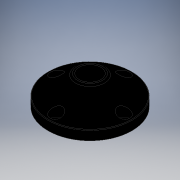
# Autodesk Inventor part: Base
Saved by Autodesk Inventor 2017 (Build 210142000, 142)
## iProperties
Created: 2020-05-28
Part Number: Base
Material: Generic
Document SubType Name: Modeling
Designer: Sid
Density: 1 g/cm^3
Appearance: Default
Author: Sid
Autodesk Inventor part; units mm, degrees
ref_plane "YZ Plane" through (0, 0, 0) normal (1, 0, 0) x (0, 1, 0)
ref_plane "XZ Plane" through (0, 0, 0) normal (0, 1, 0) x (-1, 0, 0)
ref_plane "XY Plane" through (0, 0, 0) normal (0, 0, 1) x (1, 0, 0)
sketch "Sketch1" plane through (0, 0, 0) normal (0, 0, 1) x (1, 0, 0)
  circle A0 centre (0, 0) radius 35
  dimension "d0" = 70
  constraints: 1 centre point, 1 coincident
  measures "d0" diameter of A0
extrude "Extrusion1" add sketch "Sketch1" along normal blind 8
sketch "Sketch2" plane through (0, 0, 0) normal (1, 0, 0) x (0, 1, 0)
  line L0 (11.5, 24) -> (-11.5, 24)
  line L1 (35, 0) -> (35, 8) projected
  arc A0 (11.5, 24) -> (35, 8) centre (38.1181, 37.8375) ccw
  line L2 (35, 8) -> (-35, 8) projected
  arc A1 (-35, 8) -> (-11.5, 24) centre (-38.1181, 37.8375) ccw
  line L3 (35, 8) -> (0, 8)
  line L4 (0, 24) -> (0, 8)
  line L5 (-35, 0) -> (35, 0) projected
  point P0 (0, 0)
  dimension "d3" = 23
  dimension "d4" = 11.5
  dimension "d5" = 30
  dimension "d6" = 30
  dimension "d14" = 24
  constraints: 6 end point, 4 point on circle, 2 centre point, 2 midpoint, 1 horizontal, 1 point on line
  measures "d3" distance of L0.start L0.end
  measures "d4" horizontal distance of L0.start point (0, 0)
  measures "d5" radius of A0
  measures "d6" radius of A1
  measures "d14" distance between parallel lines of L0 L5
revolve "Revolution1" add sketch "Sketch2" angle 360 about axis through (0, 0, 24) along (0, 0, -1) contours L4 L2 A1 L0
sketch "Sketch3" plane through (0, 0, 24) normal (0, 0, 1) x (1, 0, 0)
  circle A0 centre (0, 0) radius 7.25
  dimension "d8" = 14.5
  constraints: 1 centre point, 1 coincident
  measures "d8" diameter of A0
extrude "Extrusion2" cut sketch "Sketch3" against normal through all
sketch "Sketch4" plane through (0, 0, 24) normal (0, 0, 1) x (1, 0, 0)
  circle A0 centre (0, 0) radius 9
  dimension "d11" = 18
  constraints: 1 centre point, 1 coincident
  measures "d11" diameter of A0
extrude "Extrusion3" cut sketch "Sketch4" against normal blind 21
sketch "Sketch5" plane through (0, 0, 0) normal (0, 0, -1) x (-1, 0, 0)
  circle A0 centre (0, 0) radius 28.25
  circle A1 centre (0, 28.25) radius 2.75
  circle A2 centre (-28.25, 0) radius 2.75
  circle A3 centre (0, -28.25) radius 2.75
  circle A4 centre (28.25, 0) radius 2.75
  dimension "d15" = 56.5
  dimension "d16" = 5.5
  dimension "d19" = 360
  constraints: 4 centre point, 1 coincident, 1 vertical alignment, 11 other
  measures "d16" diameter of A1
extrude "Extrusion4" cut sketch "Sketch5" against normal through all contours A0 A4 | A0 A4 | A1 A0 | A0 A1 | A3 A0 | A0 A3 | A2 A0 | A0 A2
sketch "Sketch7" plane through (0, 0, 24) normal (0, 0, 1) x (1, 0, 0)
  circle A0 centre (-28.25, 0) radius 2.75 projected
  circle A1 centre (-28.25, 0) radius 5
  circle A2 centre (0, 28.25) radius 2.75 projected
  circle A3 centre (0, 28.25) radius 5
  circle A4 centre (28.25, 0) radius 2.75 projected
  circle A5 centre (28.25, 0) radius 5
  circle A6 centre (0, -28.25) radius 2.75 projected
  circle A7 centre (0, -28.25) radius 5
  point P0 (0, 0)
  dimension "d27" = 10
  dimension "d28" = 10
  dimension "d29" = 10
  dimension "d30" = 10
  constraints: 4 centre point, 4 coincident
  measures "d27" diameter of A1
  measures "d28" diameter of A3
  measures "d29" diameter of A5
  measures "d30" diameter of A7
extrude "Extrusion5" cut sketch "Sketch7" against normal blind 21
fillet "Fillet1" radius 2 1 edges at (0, 11.5, 24)
fillet "Fillet2" radius 0.5 2 edges at (-24.7487, 24.7487, 8) (24.7487, -24.7487, 8)
equation "\"d4\" = 0.5 * d3"
equation "\"d6\" = d5"
equation "\"d28\" = d27"
equation "\"d29\" = d28"
equation "\"d30\" = d27"
body "Solid1"
